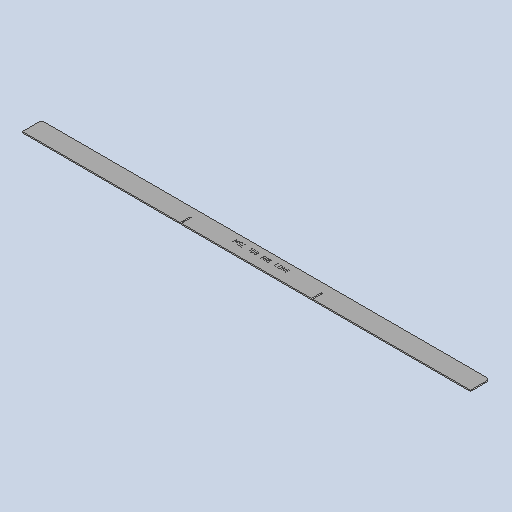
# Autodesk Inventor part: MSC 108 RIB CONE
Saved by Autodesk Inventor 2025 (Build 290162010, 162A)
## iProperties
Created: 2024-06-26
Part Number: MSC 108 RIB CONE
Material: Stainless Steel
Document SubType Name: Sheet Metal
Designer: pokla
Density: 8 g/cm^3
Sheet Metal Rule: AISI304 3mm Die 32
Appearance: Default
Stock Number: МОО 108 шпангоут конус
Mass: 1399.27 g
Surface Area: 1242.17 cm^2
Volume: 174.908 cm^3
Flat Pattern Width: 5 cm
Flat Pattern Length: 117 cm
Flat Pattern Area: 585 cm^2
Sheet Metal Width: 50,000 mm
Sheet Metal Length: 1170,000 mm
Sheet Metal Area: 58500,000 mm^2
Author: pokla
Autodesk Inventor part; units mm, degrees
ref_plane "YZ Plane" through (0, 0, 0) normal (1, 0, 0) x (0, 1, 0)
ref_plane "XZ Plane" through (0, 0, 0) normal (0, 1, 0) x (-1, 0, 0)
ref_plane "XY Plane" through (0, 0, 0) normal (0, 0, 1) x (1, 0, 0)
sketch "Sketch1" plane through (0, 0, 0) normal (0, 0, 1) x (1, 0, 0)
  line L0 (-585, 50) -> (585, 50)
  line L1 (585, 50) -> (585, 0)
  line L2 (585, 0) -> (-585, 0)
  line L3 (-585, 0) -> (-585, 50)
  circle A0 centre (-585, 0) radius 25
  circle A1 centre (585, 0) radius 25
  line L4 (585, 0) -> (642.2042, 48)
  line L5 (642.2042, 48) -> (642.2042, 50)
  line L6 (642.2042, 50) -> (585, 50)
  point P0 (0, 0)
  point P1 (0, 0)
  point P2 (-585, 25)
  point P3 (-560, 0)
  point P4 (560, 0)
  point P5 (585, 25)
  point P6 (604.1511, 16.0697)
  dimension "d16" = 50
  dimension "d17" = 1170
  dimension "d18" = 50
  dimension "d19" = 50
  dimension "d32" = 2
  dimension "d33" = 50
  measures "d16" distance of L0.end L1.end
  measures "d17" distance of L0.start L0.end
  measures "d18" diameter of A0
  measures "d19" diameter of A1
  measures "d32" distance of L4.end L5.end
  measures "d33" angle of L1 L4
extrude "Plate2" add sketch "Sketch1" against normal blind 3 contours L0 L1 A1 L2 A0 L3 | A0 L2 L3 | L1 L2 A1 picked at (-583.1457, 16.4577)
sketch "Sketch2" plane through (0, 0, 0) normal (0, 0, 1) x (1, 0, 0)
  line L0 (-585, 0) -> (585, 0) projected
  line L1 (585, 50) -> (-585, 50) projected
  line L2 (-171.55, 26) -> (-171.55, 202.9149) construction
  line L3 (-173.1, 26) -> (-170, 26)
  line L4 (-170, 26) -> (-170, 0)
  line L5 (-170, 0) -> (-173.1, 0)
  line L6 (-173.1, 0) -> (-173.1, 26)
  line L7 (171.55, 26) -> (171.55, 202.9149) construction
  line L8 (170, 0) -> (173.1, 0)
  line L9 (173.1, 0) -> (173.1, 26)
  line L10 (173.1, 26) -> (170, 26)
  line L11 (170, 26) -> (170, 0)
  line L12 (0, 236.7146) -> (0, 0) construction
  point P0 (0, 0)
  point P1 (170, 0)
  point P2 (173.1, 0)
  point P3 (-173.1, 0)
  point P4 (-170, 0)
  dimension "d39" = 26
  dimension "d41" = 3.1
  dimension "d43" = 340
  constraints: 22 end point, 4 midpoint, 4 parallel, 3 perpendicular, 2 collinear, 2 equal length, 2 horizontal, 1 vertical, 1 other
  measures "d39" distance of L4.start L4.end
  measures "d41" distance of L4.end L5.end
  measures "d43" distance between parallel lines of L11 L4
extrude "Extrusion1" cut sketch "Sketch2" against normal through all
sketch "Sketch4" plane through (0, 0, 0) normal (0, 0, 1) x (1, 0, 0)
  line L0 (-62.2268, 17.4688) -> (-62.2268, 36.055) construction
  line L1 (-62.2268, 36.055) -> (82.8811, 36.055) construction
  line L2 (82.8811, 36.055) -> (82.8811, 17.4688) construction
  line L3 (82.8811, 17.4688) -> (-62.2268, 17.4688) construction
  point P0 (0, 0)
  constraints: 2 other
mark "Mark1"
chamfer "Corner Chamfer1" distance 6 angle 45 2 edges at (585, 50, -1.5) (-585, 50, -1.5)
equation "\"d20\" = Thickness"
equation "\"BendReliefWidth\" = Thickness"
equation "\"BendReliefDepth\" = 0.5 * Thickness"
equation "\"CornerReliefSize\" = 4 * Thickness"
equation "\"MinimumRemnant\" = 2 * Thickness"
equation "\"TransitionRadius\" = BendRadius"
equation "\"JacobiRadiusSize\" = BendRadius"
equation "\"GapSize\" = Thickness"
equation "\"Thickness\" = 3"
equation "\"BendRadius\" = 5"
body "Solid2"
